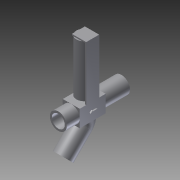
# Autodesk Inventor part: solenoid valve
Saved by Autodesk Inventor 2011 (Build 150239000, 239)
## iProperties
Created: 2013-11-19
Part Number: solenoid valve
Document SubType Name: Modeling
Designer: Devon
Density: 1 g/cm^3
Author: Devon
Autodesk Inventor part; units mm, degrees
ref_plane "YZ Plane" through (0, 0, 0) normal (1, 0, 0) x (0, 1, 0)
ref_plane "XZ Plane" through (0, 0, 0) normal (0, 1, 0) x (-1, 0, 0)
ref_plane "XY Plane" through (0, 0, 0) normal (0, 0, 1) x (1, 0, 0)
sketch "Sketch1" plane through (0, 0, 0) normal (0, 0, 1) x (1, 0, 0)
  circle A0 centre (0, 0) radius 6.35
  circle A1 centre (0, 0) radius 8.2824
  dimension "d0" = 12.7
  constraints: 2 centre point, 2 coincident
  measures "d0" diameter of A0
extrude "Extrusion1" add sketch "Sketch1" along normal blind 23.8125
sketch "Sketch2" plane through (0, 0, 23.8125) normal (0, 0, 1) x (1, 0, 0)
  circle A0 centre (0, 0) radius 6.35 projected
  circle A1 centre (0, 0) radius 8.2824 projected
  line L0 (8.2824, 8.2824) -> (-8.2824, 8.2824)
  line L1 (-8.2824, -8.2824) -> (8.2824, -8.2824)
  line L2 (8.2824, -8.2824) -> (8.2824, 8.2824)
  line L3 (-8.2824, 8.2824) -> (-8.2824, -8.2824)
  circle A2 centre (0, 0) radius 6.35
  constraints: 8 end point, 2 parallel, 1 centre point, 1 coincident, 1 concentric, 1 horizontal
extrude "Extrusion2" add sketch "Sketch2" along normal blind 25.4
sketch "Sketch3" plane through (0, 0, 49.2125) normal (0, 0, 1) x (1, 0, 0)
  circle A0 centre (0, 0) radius 6.35 projected
  circle A1 centre (0, 0) radius 6.35
  circle A2 centre (0, 0) radius 8.2824
  constraints: 2 centre point, 2 coincident, 1 concentric
extrude "Extrusion3" add sketch "Sketch3" along normal blind 12.7
sketch "Sketch4" plane through (8.2824, -8.2824, 23.8125) normal (1, 0, 0) x (0, 0, -1)
  line L0 (-15.8821, 8.2824) -> (-14.086, 10.0784)
  line L1 (-15.8821, 8.2824) -> (-13.3421, 8.2824) construction
  line L2 (-14.086, 10.0784) -> (-14.086, 9.1804)
  line L3 (-15.8821, 8.2824) -> (-14.086, 6.4863)
  line L4 (-14.086, 6.4863) -> (-14.086, 7.3843)
  line L5 (-14.086, 7.3843) -> (-9.4174, 7.3843)
  line L6 (-9.4174, 7.3843) -> (-9.4174, 9.1804)
  line L7 (-9.4174, 9.1804) -> (-14.086, 9.1804)
  point P0 (23.8125, 8.2824)
  dimension "d7" = 2.54
  dimension "d8" = 45
  constraints: 16 end point, 2 perpendicular, 1 equal length, 1 horizontal
  measures "d7" distance of L0.start L0.end
  measures "d8" angle of L1 L0
extrude "Extrusion4" add sketch "Sketch4" along normal blind 1.27
sketch "Sketch5" plane through (0, 8.2824, 23.8125) normal (0, 1, 0) x (1, 0, 0)
  circle A0 centre (0, -12.7) radius 4.1412
  point P0 (0, 23.8125)
  constraints: 1 centre point
extrude "Extrusion5" add sketch "Sketch5" along normal blind 1.27
sketch "Sketch6" plane through (0, 9.5524, 36.5125) normal (0, 1, 0) x (1, 0, 0)
  circle A0 centre (0, 0) radius 4.1412 projected
  circle A1 centre (0, 0) radius 7.62
  point P0 (0, 36.5125)
  dimension "d13" = 15.24
  constraints: 1 centre point, 1 coincident
  measures "d13" diameter of A1
extrude "Extrusion6" add sketch "Sketch6" along normal blind 50.8 contours A0 | A1
sketch "Sketch7" plane through (0, 8.2824, 23.8125) normal (0, 1, 0) x (1, 0, 0)
  line L0 (8.2824, 0) -> (8.2824, -25.4) projected
  line L1 (8.2824, -19.0619) -> (8.2824, -6.3591)
  line L2 (8.2824, -6.3591) -> (7.0124, -6.3591)
  line L3 (7.0124, -6.3591) -> (7.0124, -19.0619)
  line L4 (7.0124, -19.0619) -> (8.2824, -19.0619)
  point P0 (0, 23.8125)
  dimension "d16" = 1.27
  constraints: 8 end point, 2 perpendicular, 2 point on line, 1 parallel
  measures "d16" distance of L1.end L2.end
extrude "Extrusion7" add sketch "Sketch7" along normal blind 53.34
sketch "Sketch8" plane through (7.0124, 8.2824, 30.1716) normal (-1, 0, 0) x (0, 0, 1)
  line L0 (12.7028, 0) -> (12.7028, 53.34) projected
  line L1 (0, 53.34) -> (12.7028, 53.34)
  line L2 (12.7028, 53.34) -> (12.7028, 52.07)
  line L3 (12.7028, 52.07) -> (0, 52.07)
  line L4 (0, 52.07) -> (0, 53.34)
  point P0 (-30.1716, -8.2824)
  dimension "d19" = 1.27
  constraints: 8 end point, 2 parallel, 1 horizontal, 1 perpendicular, 1 point on line
  measures "d19" distance of L1.end L2.end
extrude "Extrusion8" add sketch "Sketch8" along normal blind 12.7
sketch "Sketch9" plane through (-8.2824, -8.2824, 23.8125) normal (0, -1, 0) x (1, 0, 0)
  line L0 (0, 0) -> (0, 25.4) projected
  line L1 (16.5647, 0) -> (16.5647, 25.4) projected
  circle A0 centre (8.2824, 12.7) radius 8.2824
  line L2 (0, 21.8506) -> (16.5647, 21.8506)
  point P0 (8.2824, -23.8125)
  constraints: 2 end point, 2 point on line, 1 centre point, 1 perpendicular
revolve "Revolution1" add sketch "Sketch9" angle 45 about axis through (-8.2824, -8.2824, 45.6631) along (-1, 0, 0) contours A0
sketch "Sketch10" plane through (0, -14.7528, 39.1926) normal (0, -0.7071068, 0.7071068) x (-1, 0, 0)
  circle A0 centre (0, 0) radius 8.2824 projected
  circle A1 centre (0, 0) radius 8.2824
  point P0 (0, 17.2816)
  constraints: 1 centre point, 1 coincident, 1 concentric
extrude "Extrusion9" add sketch "Sketch10" along normal blind 25.4
body "Solid1"
